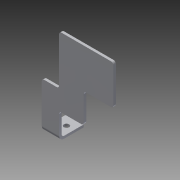
# Autodesk Inventor part: cylinder mount
Saved by Autodesk Inventor 2013 (Build 170138000, 138)
## iProperties
Created: 2013-02-08
Part Number: cylinder mount
Material: Aluminum 6061
Document SubType Name: Sheet Metal
Designer: Arpan
Density: 2.71 g/cm^3
Sheet Metal Rule: Default
Mass: 56.9603 g
Surface Area: 148.042 cm^2
Volume: 21.0186 cm^3
Author: Arpan
Autodesk Inventor part; units mm, degrees
ref_plane "YZ Plane" through (0, 0, 0) normal (1, 0, 0) x (0, 1, 0)
ref_plane "XZ Plane" through (0, 0, 0) normal (0, 1, 0) x (-1, 0, 0)
ref_plane "XY Plane" through (0, 0, 0) normal (0, 0, 1) x (1, 0, 0)
sketch "Sketch1" plane through (0, 0, 0) normal (0, 0, 1) x (1, 0, 0)
  line L0 (22.225, 50.8) -> (47.625, 50.8)
  line L1 (22.225, 0) -> (22.225, 50.8)
  line L2 (22.225, 0) -> (0, 0)
  line L3 (0, -59.055) -> (0, 0)
  line L4 (0, -59.055) -> (22.225, -59.055)
  line L5 (22.225, -25.4) -> (22.225, -59.055)
  line L6 (53.975, 19.05) -> (53.975, 44.45)
  line L7 (22.225, -25.4) -> (53.975, -25.4)
  line L8 (53.975, -25.4) -> (53.975, 19.05)
  line L9 (47.625, 50.8) -> (53.975, 50.8)
  line L10 (53.975, 50.8) -> (53.975, 44.45)
  point P0 (3.175, -63.5)
extrude "Plate1" add sketch "Sketch1" along normal blind 3.175
sketch "Sketch2" plane through (0, -55.88, 3.175) normal (0, -1, 0) x (1, 0, 0)
  line L0 (22.225, 0) -> (0, 0)
  line L1 (0, 0) -> (0, -31.75)
  line L2 (0, -31.75) -> (22.225, -31.75)
  line L3 (22.225, -31.75) -> (22.225, 0)
  constraints: 6 end point, 1 horizontal, 1 perpendicular, 1 vertical
edge flange "Flange1" height 31.75 angle 90 thickness 3.175 bend radius 3.175 thickness toward (0, -1, 0) relief tear relief width 3.175 relief depth 1.5875 edges at (11.1125, -59.055, 0) wall of the first edge with corners at (22.225, -55.88, 3.175) (0, -55.88, 3.175) (0, -55.88, -28.575) (22.225, -55.88, -28.575)
bend "Bend1"
corner "Corner1"
sketch "Sketch3" plane through (0, -55.88, -28.575) normal (0, 1, 0) x (1, 0, 0)
  circle A0 centre (12.7, -12.7) radius 3.3782 projected
  point P0 (0, -28.575)
extrude "Cut1" cut sketch "Sketch3" against normal blind 3.175
sketch "Sketch5" plane through (53.975, -25.4, 0) normal (1, 0, 0) x (0, 0, -1)
  line L0 (-3.175, 76.2) -> (-3.175, 0) projected
  line L1 (0, 76.2) -> (0, 0) projected
  line L2 (0, 76.2) -> (-3.175, 76.2) projected
  line L3 (-3.175, 76.2) -> (-3.175, 38.1)
  line L4 (-3.175, 38.1) -> (0, 38.1)
  point P0 (0, 25.4)
  dimension "d13" = 38.1
  constraints: 4 end point, 2 midpoint
  measures "d13" distance of L0.start L3.end
extrude "Extrusion1" add sketch "Sketch5" along normal blind 38.1
sketch "Sketch6" plane through (22.225, 50.8, 3.175) normal (0, 1, 0) x (1, 0, 0)
  line L0 (0, 0) -> (69.85, 0) projected
  line L1 (69.85, 3.175) -> (69.85, 0) projected
  line L2 (0, 3.175) -> (69.85, 3.175) projected
  line L3 (0, 3.175) -> (0, 0) projected
  point P0 (-22.225, 3.175)
extrude "Extrusion2" add sketch "Sketch6" along normal blind 12.7
fillet "Fillet2" radius 3.175 8 edges at (22.225, 63.5, 1.5875) (92.075, 63.5, 1.5875) (22.225, 0, 1.5875) (0, 0, 1.5875) (92.075, 12.7, 1.5875) (53.975, 12.7, 1.5875) (53.975, -25.4, 1.5875) (22.225, -25.4, 1.5875)
equation "\"d11\" = Thickness"
equation "\"d1\" = BendReliefWidth"
equation "\"d2\" = BendReliefDepth"
equation "\"d3\" = MinimumRemnant"
equation "\"d4\" = BendRadius"
equation "\"d7\" = BendRadius"
equation "\"d8\" = CornerReliefSize"
equation "\"d9\" = GapSize"
equation "\"d10\" = JacobiRadiusSize"
equation "\"BendRadius\" = Thickness"
equation "\"BendReliefWidth\" = Thickness"
equation "\"BendReliefDepth\" = 0.5 * Thickness"
equation "\"CornerReliefSize\" = 4 * Thickness"
equation "\"MinimumRemnant\" = 2 * Thickness"
equation "\"TransitionRadius\" = BendRadius"
equation "\"JacobiRadiusSize\" = Thickness"
equation "\"GapSize\" = Thickness"
equation "\"d0\" = BendRadius"
equation "\"Thickness\" = 3.175"
body "Solid1"
